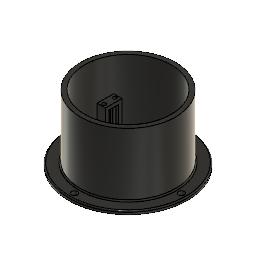
Base_v16 (Autodesk Fusion 360 design; units mm, degrees)
Autodesk Fusion 360 part; units mm, degrees
sketch "Sketch1" plane through (0, 0, 0) normal (0, 0, 1) x (1, 0, 0)
  circle A0 centre (0, 0) radius 50
  line L0 (-11.6841, 9.8041) -> (-30.6418, 25.7115)
  line L1 (-11.6841, -9.8041) -> (-30.6418, -25.7115)
  line L2 (-11.6841, 9.8041) -> (-11.6841, -9.8041)
  line L3 (-21.1841, -8.6377) -> (-33.111, -18.6456)
  arc A1 (-33.111, 18.6456) -> (-33.111, -18.6456) centre (0, 0) ccw
  line L4 (-21.1841, 8.6377) -> (-33.111, 18.6456)
  line L5 (-21.1841, 8.6377) -> (-21.1841, -8.6377)
  line L6 (-19, 7) -> (-12, 7)
  line L7 (-12, 7) -> (-12, -7)
  line L8 (-12, -7) -> (-19, -7)
  line L9 (-19, -7) -> (-19, 7)
  line L10 (-19, 7) -> (-12, -7) construction
  line L11 (-12, 7) -> (-19, -7) construction
  line L12 (30, 0) -> (30, 10)
  line L13 (30, 0) -> (30, -9)
  line L14 (30, -9) -> (38.9744, -9)
  line L15 (30, 10) -> (38.7298, 10)
  arc A2 (-30.6418, -25.7115) -> (38.9744, -9) centre (0, 0) ccw
  arc A3 (38.7298, 10) -> (-30.6418, 25.7115) centre (0, 0) ccw
  circle A4 centre (-15.5, 4.5) radius 1.5
  circle A5 centre (0, 45) radius 2.5
  circle A6 centre (-45, 0) radius 2.5
  circle A7 centre (0, -45) radius 2.5
  circle A8 centre (45, 0) radius 2.5
  circle A9 centre (33, 4.5) radius 1.5
  circle A10 centre (33, -4.5) radius 1.5
  circle A11 centre (-15.5, -4.5) radius 1.5
  point P0 (-15.5, 0)
  dimension "d30" = 3
  dimension "d32" = 5
  dimension "d34" = 360
  dimension "d36" = 3
  dimension "d45" = 3
  dimension "d46" = 3
  constraint vertical L2
  constraint horizontal L6
  constraint perpendicular L6 L7
  constraint parallel L6 L8
  constraint parallel L7 L9
  constraint coincident L10 P0
  constraint coincident L11 P0
  constraint vertical L12
  constraint parallel L12 L13
  constraint perpendicular L12 L14
  constraint coincident L15.end A2
  constraint perpendicular L12 L15
  constraint concentric A2 A3
  measures "d30" diameter of A4
  measures "d32" diameter of A5
  measures "d36" diameter of A9
  measures "d45" diameter of A11
  measures "d46" diameter of A10
extrude "Extrude1" add sketch "Sketch1" along normal blind 3 contours A0
extrude "Extrude2" add sketch "Sketch1" along normal blind 40 contours L6 L7 L8 L9
sketch "Sketch2" plane through (0, 0, 0) normal (0, 0, 1) x (1, 0, 0)
  circle A0 centre (0, 0) radius 40
  dimension "d18" = 80
  constraint coincident A0.centre origin
  measures "d18" diameter of A0
sketch "Sketch3" plane through (-12, 0, 0) normal (1, 0, 0) x (0, 1, 0)
  line L0 (-7, 3) -> (7, 3)
  line L1 (7, 3) -> (7, 40)
  line L2 (7, 40) -> (-7, 40)
  line L3 (-7, 40) -> (-7, 3)
  line L4 (-4, 37) -> (4, 37)
  line L5 (4, 37) -> (4, 4.9265)
  line L6 (4, 4.9265) -> (-4, 4.9265)
  line L7 (-4, 4.9265) -> (-4, 37)
  line L8 (-4, 37) -> (4, 4.9265) construction
  line L9 (4, 37) -> (-4, 4.9265) construction
  point P0 (0, 20.9633)
  constraint horizontal L4
  constraint perpendicular L4 L5
  constraint parallel L4 L6
  constraint parallel L5 L7
  constraint coincident L8 P0
  constraint coincident L9 P0
extrude "Extrude3" cut sketch "Sketch3" against normal blind 20 contours L4 L5 L6 L7
extrude "Extrude4" add sketch "Sketch2" along normal blind 56 thin wall 3.75 inside
sketch "Sketch4" plane through (-19, 0, 0) normal (-1, 0, 0) x (0, -1, 0)
  line L0 (-4, 4.9265) -> (-4, 37)
  line L1 (-4, 37) -> (4, 37)
  line L2 (4, 37) -> (4, 4.9265)
  line L3 (4, 4.9265) -> (-4, 4.9265)
  line L4 (-7, 3) -> (7, 3)
  line L5 (7, 3) -> (7, 40)
  line L6 (7, 40) -> (-7, 40)
  line L7 (-7, 40) -> (-7, 3)
extrude "Extrude5" add 1 faces at (32.5771, 8.6653, 3) along direction (0, 0, 1) blind 37
sketch "Sketch6" plane through (0, 0, 0) normal (0, 0, 1) x (1, 0, 0)
extrude "Extrude7" add 1 faces at (32.5771, 8.6653, 40) along direction (0, 0, -1) blind 3
sketch "Sketch7" plane through (0, 0, 0) normal (1, 0, 0) x (0, 1, 0)
  circle A0 centre (0.0873, 13.0722) radius 3.75
  dimension "d39" = 7.5
  measures "d39" diameter of A0
extrude "Extrude8" cut sketch "Sketch7" against normal blind 70
fillet "Fillet1" radius 1 1 edges at (-46.6164, -18.0808, 3)
chamfer "Chamfer1" distance 1 angle 45 1 edges at (-37.2931, 14.4646, 3)
component "base" placed x (1, 0, 0) y (0, 1, 0) z (0, 0, 1) at (0, 0, 0)
